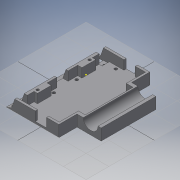
# Autodesk Inventor part: mini
Saved by Autodesk Inventor 2016 (Build 200138000, 138)
## iProperties
Created: 2016-01-06
Part Number: mini
Material: Generic
Document SubType Name: Modeling
Designer: cemer
Density: 1 g/cm^3
Appearance: Default
Mass: 33.7015 g
Surface Area: 229.203 cm^2
Volume: 33.7015 cm^3
Author: cemer
Autodesk Inventor part; units mm, degrees
ref_plane "YZ Plane" through (0, 0, 0) normal (1, 0, 0) x (0, 1, 0)
ref_plane "XZ Plane" through (0, 0, 0) normal (0, 1, 0) x (-1, 0, 0)
ref_plane "XY Plane" through (0, 0, 0) normal (0, 0, 1) x (1, 0, 0)
sketch "Sketch1" plane through (0, 0, 0) normal (0, 1, 0) x (-1, 0, 0)
  line L0 (-50.8, 50.8) -> (50.8, 50.8)
  line L1 (50.8, 50.8) -> (50.8, -50.8)
  line L2 (50.8, -50.8) -> (-50.8, -50.8)
  line L3 (-50.8, -50.8) -> (-50.8, 50.8)
  line L4 (-50.8, 50.8) -> (50.8, -50.8) construction
  line L5 (50.8, 50.8) -> (-50.8, -50.8) construction
  point P0 (0, 0)
  dimension "d0" = 101.6
  dimension "d1" = 101.6
  constraints: 12 end point, 2 midpoint, 2 parallel, 1 horizontal, 1 perpendicular
  measures "d0" distance of L1.end L2.end
  measures "d1" distance of L0.end L1.end
extrude "Extrusion1" add sketch "Sketch1" along normal blind 25.4
sketch "Sketch2" plane through (0, 25.4, 0) normal (0, 1, 0) x (1, 0, 0)
  line L0 (-50.8, -50.8) -> (50.8, -50.8) projected
  line L1 (50.8, -50.8) -> (20.32, -50.8)
  line L2 (20.32, -50.8) -> (20.32, -30.48)
  line L3 (20.32, -30.48) -> (50.8, -30.48)
  line L4 (50.8, -30.48) -> (50.8, -50.8)
  line L5 (50.8, -50.8) -> (50.8, 50.8) projected
  line L6 (50.8, 50.8) -> (20.32, 50.8)
  line L7 (20.32, 50.8) -> (20.32, 30.48)
  line L8 (20.32, 30.48) -> (50.8, 30.48)
  line L9 (50.8, 30.48) -> (50.8, 50.8)
  point P0 (0, 0)
  dimension "d4" = 30.48
  dimension "d5" = 20.32
  dimension "d6" = 20.32
  constraints: 16 end point, 4 parallel, 2 horizontal, 2 perpendicular
  measures "d4" distance of L2.end L3.end
  measures "d5" distance of L1.end L2.end
  measures "d6" distance of L7.end L6.end
extrude "Extrusion2" cut sketch "Sketch2" against normal blind 46.0375
sketch "Sketch3" plane through (50.8, 25.4, -30.48) normal (0, 0, -1) x (-1, 0, 0)
  circle A0 centre (15.24, -12.7) radius 8.255
  line L0 (30.48, -25.4) -> (0, -25.4) projected
  point P0 (50.8, -25.4)
  dimension "d9" = 16.51
  dimension "d10" = 12.7
  constraints: 1 centre point
  measures "d9" diameter of A0
  measures "d10" distance from line of L0 A0.centre
extrude "Extrusion3" cut sketch "Sketch3" against normal blind 74.6125
sketch "Sketch4" plane through (0, 25.4, 0) normal (0, 1, 0) x (1, 0, 0)
  point P0 (0, 0)
sketch "Sketch5" plane through (-50.8, 0, -50.8) normal (0, 0, -1) x (-1, 0, 0)
  line L0 (0, 0) -> (-12.7, 0)
  line L1 (0, 0) -> (-71.12, 0) projected
  line L2 (-12.7, 0) -> (-18.5876, 2.3788)
  line L3 (-18.5876, 2.3788) -> (-26.4366, 26.5356)
  line L4 (-26.4366, 26.5356) -> (2.4538, 26.5356)
  line L5 (-71.12, 25.4) -> (0, 25.4) projected
  line L6 (2.4538, 26.5356) -> (0, 0)
  point P0 (-50.8, 0)
  dimension "d13" = 12.7
  dimension "d14" = 6.35
  dimension "d15" = 158
  dimension "d16" = 25.4
  dimension "d17" = 130
  constraints: 10 end point, 1 parallel, 1 point on line
  measures "d13" distance of L0.start L0.end
  measures "d14" distance of L0.end L2.end
  measures "d15" angle of L0 L2
  measures "d16" distance of L2.end L3.end
  measures "d17" angle of L2 L3
extrude "Extrusion4" cut sketch "Sketch5" against normal blind 125.4125
sketch "Sketch6" plane through (20.32, 0, -50.8) normal (0, 0, -1) x (-1, 0, 0)
  line L0 (-30.48, 25.4) -> (-30.48, 0) projected
  line L1 (-30.48, 12.7) -> (56.0377, 12.7)
  line L2 (56.0377, 12.7) -> (56.0377, 29.7001)
  line L3 (56.0377, 29.7001) -> (-30.48, 29.7001)
  line L4 (-30.48, 29.7001) -> (-30.48, 12.7)
  point P0 (20.32, 0)
  constraints: 8 end point, 2 parallel, 1 horizontal, 1 midpoint, 1 perpendicular
extrude "Extrusion5" cut sketch "Sketch6" against normal blind 196.85
sketch "Sketch7" plane through (-28.8588, 12.7, -50.8) normal (0, 1, 0) x (1, 0, 0)
  line L0 (12.7, -99.06) -> (46.99, -99.06)
  line L1 (46.99, -99.06) -> (46.99, -77.47)
  line L2 (46.99, -77.47) -> (12.7, -77.47)
  line L3 (12.7, -77.47) -> (12.7, -99.06)
  line L4 (49.1788, -101.6) -> (0, -101.6) projected
  line L5 (0, -101.6) -> (0, 0) projected
  line L6 (46.99, -2.54) -> (12.7, -2.54)
  line L7 (12.7, -2.54) -> (12.7, -24.13)
  line L8 (12.7, -24.13) -> (46.99, -24.13)
  line L9 (46.99, -24.13) -> (46.99, -2.54)
  line L10 (-9.2412, 0) -> (49.1788, 0) projected
  line L11 (2.3638, -33.655) -> (23.9538, -33.655)
  line L12 (23.9538, -33.655) -> (23.9538, -67.945)
  line L13 (23.9538, -67.945) -> (2.3638, -67.945)
  line L14 (2.3638, -67.945) -> (2.3638, -33.655)
  line L15 (56.1638, -81.28) -> (49.1788, -81.28) projected
  line L16 (56.1638, -20.32) -> (56.1638, -81.28) projected
  point P0 (28.8588, -50.8)
  dimension "d22" = 34.29
  dimension "d23" = 21.59
  dimension "d24" = 2.54
  dimension "d25" = 12.7
  dimension "d26" = 21.59
  dimension "d27" = 2.54
  dimension "d28" = 21.59
  dimension "d29" = 34.29
  dimension "d30" = 33.655
  dimension "d31" = 3.81
  dimension "d32" = 32.21
  dimension "d33" = 53.34
  constraints: 24 end point, 6 parallel, 3 horizontal, 3 perpendicular
  measures "d22" distance of L2.end L1.end
  measures "d23" distance of L1.end L0.end
  measures "d24" distance from line of L4 L0.start
  measures "d25" distance from line of L5 L2.end
  measures "d26" distance of L7.end L6.end
  measures "d27" distance between parallel lines of L10 L6
  measures "d28" distance of L12.end L13.end
  measures "d29" distance of L11.end L12.end
  measures "d30" distance between parallel lines of L13 L4
  measures "d31" distance between parallel lines of L2 L15
  measures "d32" distance from line of L16 L11.end
  measures "d33" distance between parallel lines of L8 L2
extrude "Extrusion6" cut sketch "Sketch7" against normal blind 10.16
sketch "Sketch8" plane through (-28.8588, 2.54, -50.8) normal (0, 1, 0) x (1, 0, 0)
  circle A0 centre (5.6658, -63.5) radius 1.651
  circle A1 centre (5.6658, -38.1) radius 1.651
  line L0 (2.3638, -33.655) -> (23.9538, -33.655) projected
  line L1 (2.3638, -67.945) -> (2.3638, -33.655) projected
  circle A2 centre (42.545, -5.842) radius 1.651
  line L2 (12.7, -2.54) -> (46.99, -2.54) projected
  line L3 (46.99, -2.54) -> (46.99, -24.13) projected
  circle A3 centre (17.145, -5.842) radius 1.651
  line L4 (12.7, -24.13) -> (12.7, -2.54) projected
  circle A4 centre (42.545, -95.758) radius 1.651
  line L5 (46.99, -99.06) -> (12.7, -99.06) projected
  circle A5 centre (17.145, -95.758) radius 1.651
  point P0 (28.8588, -50.8)
  dimension "d36" = 3.302
  dimension "d37" = 3.302
  dimension "d38" = 25.4
  dimension "d39" = 4.445
  dimension "d40" = 3.302
  dimension "d41" = 3.302
  dimension "d42" = 3.302
  dimension "d43" = 3.302
  dimension "d44" = 4.445
  dimension "d45" = 3.302
  dimension "d46" = 4.445
  dimension "d47" = 3.302
  dimension "d48" = 3.302
  dimension "d49" = 3.302
  constraints: 6 centre point
  measures "d36" diameter of A0
  measures "d37" diameter of A1
  measures "d38" distance of A1.centre A0.centre
  measures "d39" distance from line of L0 A1.centre
  measures "d40" distance from line of L1 A0.centre
  measures "d41" distance from line of L1 A1.centre
  measures "d42" diameter of A2
  measures "d43" distance from line of L2 A2.centre
  measures "d44" distance from line of L3 A2.centre
  measures "d45" diameter of A3
  measures "d46" distance from line of L4 A3.centre
  measures "d47" diameter of A4
  measures "d48" distance from line of L5 A4.centre
  measures "d49" diameter of A5
extrude "Extrusion7" cut sketch "Sketch8" against normal blind 21.59
sketch "Sketch9" plane through (43.815, 12.7, -30.48) normal (0, 1, 0) x (1, 0, 0)
  line L0 (6.985, -60.96) -> (0, -60.96) projected
  line L1 (6.924, 0.1032) -> (3.4925, 0.1032)
  line L2 (3.4925, 0.1032) -> (3.4925, -60.96)
  line L3 (3.4925, -60.96) -> (6.924, -60.96)
  line L4 (6.924, -60.96) -> (6.924, 0.1032)
  point P0 (-43.815, -30.48)
  constraints: 8 end point, 2 parallel, 1 horizontal, 1 midpoint, 1 perpendicular
extrude "Extrusion8" cut sketch "Sketch9" against normal blind 24.4475
sketch "Sketch10" plane through (47.3075, 12.7, 30.48) normal (1, 0, 0) x (0, 0, -1)
  line L0 (159.4685, 88.4903) -> (-103.8502, 88.4903)
  line L1 (-103.8502, 88.4903) -> (-103.8502, -114.2762)
  line L2 (-103.8502, -114.2762) -> (159.4685, -114.2762)
  line L3 (159.4685, -114.2762) -> (159.4685, 88.4903)
  point P0 (30.48, -12.7)
  constraints: 8 end point, 2 parallel, 1 horizontal, 1 perpendicular
extrude "Extrusion9" cut sketch "Sketch10" along normal blind 64.135
sketch "Sketch11" plane through (-28.8588, 12.7, -50.8) normal (0, 1, 0) x (1, 0, 0)
  line L0 (6.5068, -99.06) -> (-6.7012, -99.06)
  line L1 (-6.7012, -99.06) -> (-6.7012, -90.932)
  line L2 (-6.7012, -90.932) -> (6.5068, -90.932)
  line L3 (6.5068, -90.932) -> (6.5068, -99.06)
  line L4 (49.1788, -101.6) -> (0, -101.6) projected
  line L5 (-9.2412, -101.6) -> (-9.2412, 0) projected
  line L6 (-6.7012, -2.54) -> (6.5068, -2.54)
  line L7 (6.5068, -2.54) -> (6.5068, -10.668)
  line L8 (6.5068, -10.668) -> (-6.7012, -10.668)
  line L9 (-6.7012, -10.668) -> (-6.7012, -2.54)
  line L10 (-3.3536, 0) -> (0, 0) projected
  point P0 (28.8588, -50.8)
  dimension "d56" = 13.208
  dimension "d57" = 8.128
  dimension "d59" = 10.668
  dimension "d60" = 2.54
  dimension "d61" = 8.128
  dimension "d62" = 2.54
  constraints: 16 end point, 4 parallel, 2 horizontal, 2 perpendicular
  measures "d56" distance of L1.end L2.end
  measures "d57" distance of L2.end L0.start
  measures "d59" distance from line of L4 L2.end
  measures "d60" distance from line of L5 L0.end
  measures "d61" distance of L6.end L7.end
  measures "d62" distance from line of L10 L6.start
extrude "Extrusion10" cut sketch "Sketch11" against normal blind 12.065
sketch "Sketch12" plane through (-28.8588, 0.635, -50.8) normal (0, 1, 0) x (1, 0, 0)
  circle A0 centre (4.8558, -94.996) radius 1.143
  line L0 (6.5068, -90.932) -> (6.5068, -99.06) projected
  circle A1 centre (4.8558, -6.604) radius 1.143
  line L1 (-6.7012, -2.54) -> (6.5068, -2.54) projected
  line L2 (0, -90.932) -> (0, -10.668) projected
  line L3 (-6.7012, -2.54) -> (0, -2.54)
  line L4 (0, -2.54) -> (0, -10.668)
  line L5 (0, -10.668) -> (-6.7012, -10.668)
  line L6 (-6.7012, -10.668) -> (-6.7012, -2.54)
  line L7 (0, -101.6) -> (0, -99.06) projected
  line L8 (0, -99.06) -> (-6.7012, -99.06)
  line L9 (-6.7012, -99.06) -> (-6.7012, -90.932)
  line L10 (-6.7012, -90.932) -> (0, -90.932)
  line L11 (0, -90.932) -> (0, -99.06)
  point P0 (28.8588, -50.8)
  dimension "d65" = 2.286
  dimension "d66" = 1.651
  dimension "d67" = 2.286
  constraints: 16 end point, 4 parallel, 2 centre point, 2 horizontal, 2 perpendicular, 1 point on line
  measures "d65" diameter of A0
  measures "d66" distance from line of L0 A0.centre
  measures "d67" diameter of A1
extrude "Extrusion11" cut sketch "Sketch12" against normal blind 26.035
sketch "Sketch13" plane through (-38.1, 0, 50.8) normal (0, 0, 1) x (1, 0, 0)
  line L0 (0, 0) -> (-0.508, 0)
  line L1 (-0.508, 0) -> (5.7329, 2.5215)
  line L2 (9.2412, 12.7) -> (15.748, 12.7) projected
  line L3 (5.7329, 2.5215) -> (9.2412, 12.7)
  line L4 (9.2412, 12.7) -> (5.8876, 2.3788) projected
  line L5 (9.2412, 12.7) -> (5.8876, 2.3788)
  line L6 (5.8876, 2.3788) -> (0, 0)
  point P0 (38.1, 0)
  dimension "d70" = 0.508
  dimension "d71" = 6.731
  dimension "d72" = 22
  constraints: 10 end point, 1 collinear, 1 horizontal
  measures "d70" distance of L0.start L0.end
  measures "d71" distance of L0.end L1.end
  measures "d72" angle of L0 L1
extrude "Extrusion12" add sketch "Sketch13" against normal blind 101.6
sketch "Sketch14" plane through (-28.8588, 0.635, -50.8) normal (0, 1, 0) x (1, 0, 0)
  line L0 (6.5068, -2.54) -> (-6.7012, -2.54)
  line L1 (-6.7012, -2.54) -> (-6.7012, -10.668)
  line L2 (-6.7012, -10.668) -> (6.5068, -10.668)
  line L3 (6.5068, -10.668) -> (6.5068, -2.54)
  line L4 (6.5068, -90.932) -> (6.5068, -99.06) projected
  line L5 (0, -90.932) -> (-6.7012, -90.932) projected
  line L6 (6.5068, -99.06) -> (-6.7012, -99.06)
  line L7 (-6.7012, -99.06) -> (-6.7012, -90.932)
  line L8 (-6.7012, -90.932) -> (6.5068, -90.932)
  line L9 (6.5068, -90.932) -> (6.5068, -99.06)
  point P0 (28.8588, -50.8)
  constraints: 16 end point, 4 parallel, 2 horizontal, 2 perpendicular
extrude "Extrusion13" cut sketch "Sketch14" along normal blind 46.0375
sketch "Sketch15" plane through (20.32, 12.7, 30.48) normal (0, 1, 0) x (1, 0, 0)
  circle A0 centre (-45.3688, 59.4741) radius 1.4986
  circle A1 centre (-45.3688, 1.4741) radius 1.4986
  line L0 (-49.1788, -9.652) -> (-49.1788, 70.612) projected
  line L1 (-49.1788, 81.28) -> (0, 81.28) projected
  point P0 (-20.32, 30.48)
  dimension "d77" = 2.9972
  dimension "d78" = 2.9972
  dimension "d79" = 58
  dimension "d80" = 3.81
  dimension "d81" = 3.81
  dimension "d82" = 21.8059
  constraints: 2 centre point
  measures "d77" diameter of A0
  measures "d78" diameter of A1
  measures "d79" distance of A1.centre A0.centre
  measures "d80" distance from line of L0 A1.centre
  measures "d81" distance from line of A0.centre L0
  measures "d82" distance from line of L1 A0.centre
extrude "Extrusion14" cut sketch "Sketch15" against normal blind 6.35
sketch "Sketch16" plane through (20.32, 12.7, 30.48) normal (0, 1, 0) x (1, 0, 0)
  line L0 (-49.1788, -9.652) -> (-42.672, -9.652) projected
  line L1 (-45.9254, -9.652) -> (-45.9254, -2.032)
  line L2 (-45.9254, -2.032) -> (-42.1154, -2.032)
  line L3 (-42.1154, -2.032) -> (-42.1154, 13.377)
  line L4 (-45.9254, -9.652) -> (-2.1888, -9.652)
  line L5 (-2.1888, 3.81) -> (-2.1888, -17.78) projected
  line L6 (-36.4788, 3.81) -> (-2.1888, 3.81) projected
  line L7 (-2.1888, 3.81) -> (5.4312, 3.81)
  line L8 (6.985, 60.96) -> (6.985, 0) projected
  line L9 (5.4312, 3.81) -> (5.4312, 57.15)
  line L10 (-2.1888, 57.15) -> (-36.4788, 57.15) projected
  line L11 (5.4312, 57.15) -> (-2.1888, 57.15)
  line L12 (-2.1888, 57.15) -> (-2.1888, 70.612)
  line L13 (-2.1888, 70.612) -> (-36.4788, 70.612)
  line L14 (-42.672, 70.612) -> (-49.1788, 70.612) projected
  line L15 (-36.4788, 70.612) -> (-42.672, 70.612)
  line L16 (-42.672, 70.612) -> (-45.9254, 70.612)
  line L17 (-45.9254, 70.612) -> (-45.9254, 62.992)
  line L18 (-45.9254, 62.992) -> (-42.1154, 62.992)
  line L19 (-42.1154, 62.992) -> (-42.1154, 47.625)
  line L20 (-46.815, 47.625) -> (-25.225, 47.625) projected
  line L21 (-42.1154, 13.377) -> (-42.1154, 47.625)
  point P0 (-20.32, 30.48)
  dimension "d85" = 7.62
  dimension "d86" = 3.81
  dimension "d87" = 7.62
  dimension "d88" = 7.62
  dimension "d89" = 3.81
  constraints: 30 end point, 10 perpendicular, 2 midpoint, 2 point on line, 1 collinear, 1 horizontal, 1 vertical
  measures "d85" distance of L1.start L1.end
  measures "d86" distance of L1.end L2.end
  measures "d87" distance of L5.start L7.end
  measures "d88" distance of L16.end L17.end
  measures "d89" distance of L17.end L18.end
extrude "Extrusion15" cut sketch "Sketch16" against normal blind 10.16
sketch "Sketch17" plane through (20.32, 12.7, 30.48) normal (0, 1, 0) x (1, 0, 0)
  line L0 (-36.4788, 70.612) -> (-36.4788, 78.74) projected
  line L1 (-42.672, 78.74) -> (-36.4788, 78.74)
  line L2 (-36.4788, 78.74) -> (-36.4788, 70.612)
  line L3 (-36.4788, 70.612) -> (-42.672, 70.612)
  line L4 (-42.672, 70.612) -> (-42.672, 78.74)
  line L5 (-36.4788, -9.652) -> (-42.672, -9.652) projected
  line L6 (-36.4788, -17.78) -> (-36.4788, -9.652) projected
  line L7 (-42.672, -9.652) -> (-36.4788, -9.652)
  line L8 (-36.4788, -9.652) -> (-36.4788, -17.78)
  line L9 (-36.4788, -17.78) -> (-42.672, -17.78)
  line L10 (-42.672, -17.78) -> (-42.672, -9.652)
  point P0 (-20.32, 30.48)
  constraints: 16 end point, 4 parallel, 2 horizontal, 2 perpendicular
extrude "Extrusion16" cut sketch "Sketch17" against normal blind 10.16
sketch "Sketch18" plane through (-26.495, 12.7, 17.145) normal (0, 1, 0) x (1, 0, 0)
  line L0 (6.4509, 23.495) -> (-27.6317, 23.495)
  line L1 (-27.6317, 23.495) -> (-27.6317, 10.795)
  line L2 (-27.6317, 10.795) -> (6.4509, 10.795)
  line L3 (6.4509, 10.795) -> (6.4509, 23.495)
  line L4 (46.815, -33.655) -> (-2.3638, -33.655) projected
  line L5 (33.1962, -36.0333) -> (20.4962, -36.0333)
  line L6 (20.4962, -36.0333) -> (20.4962, 70.9556)
  line L7 (20.4962, 70.9556) -> (33.1962, 70.9556)
  line L8 (33.1962, 70.9556) -> (33.1962, -36.0333)
  line L9 (44.6262, -9.525) -> (44.6262, -31.115) projected
  point P0 (26.495, 17.145)
  dimension "d94" = 12.7
  dimension "d95" = 44.45
  dimension "d96" = 12.7
  dimension "d97" = 11.43
  constraints: 16 end point, 4 parallel, 2 horizontal, 2 perpendicular
  measures "d94" distance of L0.end L1.end
  measures "d95" distance from line of L4 L1.end
  measures "d96" distance of L6.end L7.end
  measures "d97" distance from line of L9 L5.start
extrude "Extrusion17" cut sketch "Sketch18" against normal blind 10.16
body "Solid1"
